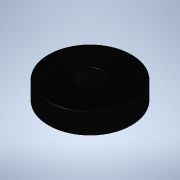
# Autodesk Inventor part: YTP-AP-E19-R1.0
Saved by Autodesk Inventor 2020.4 (Build 244396000, 396)
## iProperties
RuleStatus: InUse
AfterDocNew0: iPropertyEnforcement
BeforeDocSave0: Materialprüfung
Created: 2021-08-29
Part Number: YTP-AP-E19-R1.0
Material: Gummi
Document SubType Name: Modeling
Designer: Uwe Wieser
Mass: 0.0206898 g
Surface Area: 0.595082 cm^2
Volume: 0.0222471 cm^3
Density: 0.93 g/cm^3
Appearance: Schwarz
Project: Airbrush
Description: O-Ring-Ventil
Werkstoff: Gummi
Author: Uwe Wieser
Autodesk Inventor part; units mm, degrees
ref_plane "YZ Plane" through (0, 0, 0) normal (1, 0, 0) x (0, 1, 0)
ref_plane "XZ Plane" through (0, 0, 0) normal (0, 1, 0) x (-1, 0, 0)
ref_plane "XY Plane" through (0, 0, 0) normal (0, 0, 1) x (1, 0, 0)
sketch "Skizze1" plane through (0, 0, 0) normal (0, 0, 1) x (1, 0, 0)
  circle A0 centre (0, 0) radius 0.75
  circle A1 centre (0, 0) radius 2.5
  dimension "d0" = 1.5
  dimension "d1" = 5
  constraints: 2 centre point, 2 coincident
  measures "d0" diameter of A0
  measures "d1" diameter of A1
extrude "Extrusion1" add sketch "Skizze1" along normal mid plane 1.25
fillet "Rundung1" radius 0.1 4 edges at (-2.5, 0, 0.625) (-2.5, 0, -0.625) (-0.75, 0, 0.625) (-0.75, 0, -0.625)
